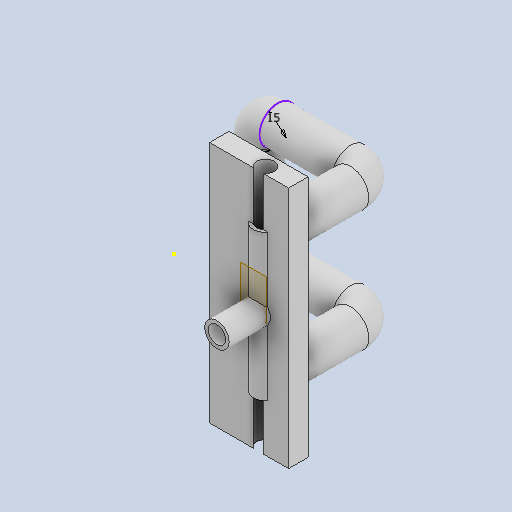
# Autodesk Inventor part: T-joint_hand
Saved by Autodesk Inventor 2025 (Build 290162000, 162)
## iProperties
Created: 2025-07-16
Part Number: T-joint_hand
Material: Generic
Document SubType Name: Modeling
Designer: Pravoslav
Density: 1 g/cm^3
Appearance: Default
Author: Pravoslav
Autodesk Inventor part; units mm, degrees
ref_plane "YZ Plane" through (0, 0, 0) normal (1, 0, 0) x (0, 1, 0)
ref_plane "XZ Plane" through (0, 0, 0) normal (0, 1, 0) x (-1, 0, 0)
sketch "Sketch1" plane through (0, 0, 0) normal (0, 1, 0) x (-1, 0, 0)
  circle A0 centre (0, 0) radius 3.575
  circle A1 centre (0, 0) radius 5
  dimension "d0" = 7.15
  dimension "d1" = 10
  constraints: 2 centre point, 2 coincident
  measures "d0" diameter of A0
  measures "d1" diameter of A1
extrude "Extrusion1" add sketch "Sketch1" along normal mid plane 60
ref_plane "Work Plane1" through (0, 0, 5) normal (0, 0, 1) x (1, 0, 0)
sketch "Sketch2" plane through (0, 0, 5) normal (0, 0, 1) x (1, 0, 0)
  circle A0 centre (0, 0) radius 3.575
  circle A1 centre (0, 0) radius 5
  line L0 (5, 30) -> (-5, 30) projected
  dimension "d4" = 7.15
  dimension "d5" = 10
  dimension "d22" = 0
  constraints: 2 centre point, 1 coincident
  measures "d4" diameter of A0
  measures "d5" diameter of A1
  measures "d22" distance of point (0, 0) A0.centre
extrude "Extrusion2" add sketch "Sketch2" along normal blind 15 and the other way blind 5
sketch "Sketch3" plane through (0, 0, 20) normal (0, 0, 1) x (1, 0, 0)
  circle A0 centre (0, 0) radius 3.575
  constraints: 1 centre point, 1 coincident
extrude "Extrusion3" cut sketch "Sketch3" against normal up to surface
sketch "Sketch4" plane through (0, 30, 0) normal (0, 1, 0) x (1, 0, 0)
  circle A0 centre (0, 0) radius 3.675
  dimension "d13" = 7.35
  constraints: 1 centre point, 1 coincident
  measures "d13" diameter of A0
extrude "Extrusion4" cut sketch "Sketch4" against normal through all
ref_plane "Work Plane3" through (0, 0, -5) normal (0, 0, 1) x (1, 0, 0)
sketch "Sketch6" plane through (0, 0, -5) normal (0, 0, 1) x (1, 0, 0)
  line L0 (12.5, -50) -> (-12.5, -50)
  line L1 (-12.5, -50) -> (-12.5, 50)
  line L2 (-12.5, 50) -> (12.5, 50)
  line L3 (12.5, 50) -> (12.5, -50)
  line L4 (12.5, -50) -> (-12.5, 50) construction
  line L5 (-12.5, -50) -> (12.5, 50) construction
  point P0 (0, 0)
  dimension "d23" = 25
  dimension "d24" = 100
  constraints: 12 end point, 2 midpoint, 2 parallel, 1 horizontal, 1 perpendicular
  measures "d23" distance between parallel lines of L1 L3
  measures "d24" distance between parallel lines of L0 L2
extrude "Extrusion6" add sketch "Sketch6" along normal blind 8
sketch "Sketch7" plane through (0, -30, 0) normal (0, -1, 0) x (1, 0, 0)
  circle A0 centre (0, 0) radius 3.615
  dimension "d27" = 7.23
  constraints: 1 centre point, 1 coincident
  measures "d27" diameter of A0
extrude "Extrusion7" cut sketch "Sketch7" along normal through all both and the other way through all
sketch "Sketch8" plane through (0, 0, -5) normal (0, 0, -1) x (-1, 0, 0)
  circle A0 centre (0, -25) radius 7.5
  circle A1 centre (0, 25) radius 7.5
  point P0 (0, 0)
  dimension "d30" = 15
  dimension "d31" = 15
  dimension "d32" = 50
  dimension "d33" = 25
  constraints: 2 centre point
  measures "d30" diameter of A0
  measures "d31" diameter of A1
  measures "d32" distance of A1.centre A0.centre
  measures "d33" distance of A0.centre point (0, 0)
extrude "Extrusion8" add sketch "Sketch8" along normal blind 30
sketch "Sketch9" plane through (0, 25, -35) normal (0, 0, -1) x (-1, 0, 0)
  circle A0 centre (0, 0) radius 7.5
  line L0 (7.5, 0) -> (7.5, -9.7245)
  line L1 (7.5, -9.7245) -> (7.5, 12.7829)
  point P0 (0, -25)
  constraints: 4 end point, 1 horizontal alignment, 1 point on line, 1 vertical, 2 other
revolve "Revolution1" add sketch "Sketch9" angle 90 about axis through (-7.5, 15.2755, -35) along (0, 1, 0)
mirror "Mirror1" about plane through (0, 0, 0) normal (0, 1, 0) of "Revolution1"
sketch "Sketch10" plane through (-7.5, 25, -42.5) normal (-1, 0, 0) x (0, 0, 1)
  circle A0 centre (0, 0) radius 7.5
  point P0 (42.5, -25)
  dimension "d37" = 15
  constraints: 1 centre point
  measures "d37" diameter of A0
extrude "Extrusion9" add sketch "Sketch10" along normal blind 30
mirror "Mirror2" about plane through (0, 0, 0) normal (0, 1, 0) of "Extrusion9"
sketch "Sketch11" plane through (-37.5, 25, -42.5) normal (-1, 0, 0) x (0, 0, 1)
  circle A0 centre (0, 0) radius 7.5
  circle A1 centre (0, 0) radius 7.5 projected
  line L0 (0, -7.5) -> (-9.6615, -7.5)
  line L1 (-9.6615, -7.5) -> (9.5932, -7.5)
  point P0 (42.5, -25)
  dimension "d40" = 15
  constraints: 4 end point, 2 horizontal, 1 centre point, 1 point on line, 1 tangent, 1 vertical alignment, 1 other
  measures "d40" diameter of A0
sketch "Sketch12" plane through (-37.5, -25, -42.5) normal (-1, 0, 0) x (0, 0, 1)
  circle A0 centre (0, 0) radius 7.5
  line L0 (0, 7.5) -> (-6.8839, 7.5)
  circle A1 centre (0, 0) radius 7.5 projected
  line L1 (-6.8839, 7.5) -> (7.5, 7.5)
  point P0 (42.5, 25)
  dimension "d41" = 15
  constraints: 4 end point, 2 horizontal, 2 vertical alignment, 1 point on line, 2 other
revolve "Revolution2" add sketch "Sketch12" angle 90 about axis through (-37.5, -17.5, -49.3839) along (0, 0, -1)
mirror "Mirror3" about plane through (0, 0, 0) normal (0, 1, 0) of "Revolution2"
sketch "Sketch13" plane through (-45, 17.5, -42.5) normal (0, -1, 0) x (1, 0, 0)
  circle A0 centre (0, 0) radius 7.5
  point P0 (45, 42.5)
  dimension "d43" = 15
  constraints: 1 centre point
  measures "d43" diameter of A0
extrude "Extrusion10" add sketch "Sketch13" along normal up to surface (35 mm away)
sketch "Sketch14" plane through (-12.5, -50, -5) normal (-1, 0, 0) x (0, 0, 1)
  line L0 (0, 100) -> (0, 0) projected
  line L1 (8, 100) -> (8, 0) projected
  line L2 (0, 0) -> (8, 0)
  line L3 (8, 0) -> (8, 100)
  line L4 (8, 100) -> (0, 100)
  line L5 (0, 100) -> (0, 0)
  point P0 (5, 50)
  constraints: 8 end point, 2 parallel, 1 horizontal, 1 perpendicular
extrude "Extrusion11" add sketch "Sketch14" along normal blind 7.5
sketch "Sketch5" plane through (0, 0, -5) normal (0, 0, 1) x (1, 0, 0)
  line L0 (5, 15) -> (-5, 15) projected
  line L1 (-5, -15) -> (5, -15) projected
  line L2 (2, 15) -> (-2, 15)
  line L3 (-2, 15) -> (-2, -15)
  line L4 (-2, -15) -> (2, -15)
  line L5 (2, -15) -> (2, 15)
  point P0 (0, 0)
  dimension "d16" = 4
  dimension "d17" = 2
  constraints: 8 end point, 2 parallel, 2 point on line, 1 horizontal, 1 perpendicular
  measures "d16" distance between parallel lines of L3 L5
  measures "d17" distance from line of point (0, 0) L5
body "Solid1"
